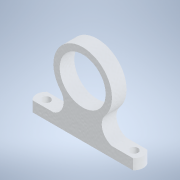
# Autodesk Inventor part: SoportePolea
Saved by Autodesk Inventor 2021 (Build 250183000, 183)
## iProperties
Created: 2022-10-28
Part Number: SoportePolea
Material: Generic
Document SubType Name: Modeling
Designer: zulet
Density: 1 g/cm^3
Appearance: White
Mass: 3.29866 g
Surface Area: 26.1546 cm^2
Volume: 3.29866 cm^3
Author: zulet
Autodesk Inventor part; units mm, degrees
ref_plane "YZ Plane" through (0, 0, 0) normal (1, 0, 0) x (0, 1, 0)
ref_plane "XZ Plane" through (0, 0, 0) normal (0, 1, 0) x (-1, 0, 0)
ref_plane "XY Plane" through (0, 0, 0) normal (0, 0, 1) x (1, 0, 0)
sketch "Sketch1" plane through (0, 0, 0) normal (0, 0, 1) x (1, 0, 0)
  circle A0 centre (0, 0) radius 4
  circle A1 centre (0, 0) radius 11
  line L0 (-25.9378, -1.7681) -> (-27.6396, -2.8187) projected
  line L1 (-27.6396, -2.8187) -> (-14.9069, -23.4452) projected
  line L2 (-14.9069, -23.4452) -> (-13.205, -22.3947) projected
  line L3 (0, 0) -> (11.913, 7.3539) construction
  circle A2 centre (0, 0) radius 14
  line L4 (-24, -20) -> (24, -20)
  line L5 (24, -20) -> (24, -25)
  line L6 (24, -25) -> (-24, -25)
  line L7 (-24, -25) -> (-24, -20)
  arc A3 (-14, -20) -> (-10.7276, -8.9954) centre (-16, -13.4164) ccw
  line L8 (-14, 0) -> (-14, -25) construction
  line L9 (0, 0) -> (-14, 0) construction
  line L10 (0, 0) -> (14, 0) construction
  line L11 (14, 0) -> (14, -25) construction
  arc A4 (10.7276, -8.9954) -> (14, -20) centre (16, -13.4164) ccw
  dimension "d0" = 8
  dimension "d1" = 22
  dimension "d19" = 3
  dimension "d20" = 25
  dimension "d21" = 5
  dimension "d22" = 2
  dimension "d23" = 2
  dimension "d24" = 10
  dimension "d25" = 10
  constraints: 18 end point, 8 point on circle, 6 point on line, 5 centre point, 3 horizontal, 3 perpendicular, 2 coincident, 2 parallel, 2 tangent, 1 vertical
  measures "d0" diameter of A0
  measures "d1" diameter of A1
  measures "d19" radial gap between concentric circles of A1 A2
  measures "d20" distance from line of L6 point (0, 0)
  measures "d21" distance of L4.end L5.end
  measures "d22" distance from line of L8 A3.centre
  measures "d23" distance from line of L11 A4.centre
  measures "d24" distance between parallel lines of L8 L7
  measures "d25" distance between parallel lines of L11 L5
extrude "Extrusion1" add sketch "Sketch1" along normal blind 7 contours A2 | A2 A4 L4 A3 | L4 L5 L6 L7
sketch "Sketch5" plane through (-24, -20, 0) normal (0, 1, 0) x (1, 0, 0)
  circle A0 centre (3, -3.5) radius 2
  circle A1 centre (45, -3.5) radius 2
  line L0 (3, -3.5) -> (45, -3.5) construction
  line L1 (0, 0) -> (0, -7) projected
  line L2 (48, 0) -> (48, -7) projected
  line L3 (10, 0) -> (0, 0) projected
  circle A2 centre (3, -3.5) radius 4.6098
  line L4 (0, 0) -> (48, 0) projected
  circle A3 centre (45, -3.5) radius 4.6098
  point P0 (24, 0)
  dimension "d26" = 4
  dimension "d27" = 4
  dimension "d28" = 3
  dimension "d29" = 3
  dimension "d30" = 3.5
  constraints: 2 centre point, 2 coincident, 2 end point, 1 horizontal, 6 other
  measures "d26" diameter of A0
  measures "d27" diameter of A1
  measures "d28" distance from line of L1 L0.start
  measures "d29" distance from line of L2 L0.end
  measures "d30" distance between parallel lines of L0 L3
extrude "Extrusion6" cut sketch "Sketch5" against normal up to surface (5 mm away) contours A0 | A1
extrude "Extrusion7" add sketch "Sketch5" against normal up to surface (5 mm away) contours L1 A2 | A3 L2
equation "\"d0\" = DIR"
equation "\"d1\" = DER"
equation "\"d20\" = HSE"
equation "\"DER\" = 22"
equation "\"HR\" = 7"
equation "\"DIR\" = 8"
equation "\"DEM\" = 4"
equation "\"Dmarc\" = 17.5"
equation "\"Bsm\" = 22.5"
equation "\"Hsm\" = 12"
equation "\"Lsm\" = 21"
equation "\"Dsc\" = 5"
equation "\"RC\" = 4"
equation "\"PB\" = 25"
equation "\"TB\" = 3"
equation "\"HSE\" = 25"
equation "\"LMaSP\" = 46.5"
body "Solid1"
